Autodesk Fusion 360 part; units mm, degrees
note: some values were not read from the file. Set by a fixed rule: which sketch regions a step uses.
(part 2 of 2)
  line L93 (-6.3283, 34.4045) -> (-6.9169, 34.9918)
  spline S105 degree 3 poles (-6.9169, 34.9918) (-6.9414, 35.0193) (-6.976, 35.0359) (-7.0129, 35.0377) knots 0 0 0 0 1 1 1 1
  spline S106 degree 3 poles (-7.0129, 35.0377) (-7.0497, 35.0395) (-7.0858, 35.0264) (-7.1129, 35.0014) knots 0 0 0 0 1 1 1 1
  spline S107 degree 3 poles (-7.1129, 35.0014) (-7.1163, 34.9983) (-7.1195, 34.9951) (-7.1225, 34.9918) knots 0 0 0 0 1 1 1 1
  spline S108 degree 3 poles (-7.1225, 34.9918) (-7.1791, 34.9347) (-7.1791, 34.8426) (-7.1225, 34.7855) knots 0 0 0 0 1 1 1 1
  line L94 (-7.1225, 34.7855) -> (-6.428, 34.0972)
  spline S109 degree 3 poles (-6.428, 33.3938) (-6.4035, 33.3662) (-6.3689, 33.3497) (-6.3321, 33.3478) knots 0 0 0 0 1 1 1 1
  spline S110 degree 3 poles (-6.3321, 33.3478) (-6.2952, 33.346) (-6.2592, 33.3591) (-6.2321, 33.3841) knots 0 0 0 0 1 1 1 1
  spline S111 degree 3 poles (-6.2321, 33.3841) (-6.2287, 33.3872) (-6.2255, 33.3904) (-6.2224, 33.3938) knots 0 0 0 0 1 1 1 1
  line L95 (-6.2224, 33.3938) -> (-5.5348, 34.0862)
  spline S112 degree 3 poles (-5.5348, 34.0862) (-5.5068, 34.1107) (-5.49, 34.1456) (-5.4882, 34.1828) knots 0 0 0 0 1 1 1 1
  spline S113 degree 3 poles (-5.4882, 34.1828) (-5.4864, 34.22) (-5.4997, 34.2563) (-5.5252, 34.2835) knots 0 0 0 0 1 1 1 1
  spline S114 degree 3 poles (-5.5252, 34.2835) (-5.5282, 34.2869) (-5.5314, 34.2901) (-5.5348, 34.2931) knots 0 0 0 0 1 1 1 1
  spline S115 degree 3 poles (-5.5348, 34.2931) (-5.5622, 34.3198) (-5.5991, 34.3344) (-5.6373, 34.3337) knots 0 0 0 0 1 1 1 1
  spline S116 degree 3 poles (-5.6373, 34.3337) (-5.6755, 34.3337) (-5.7124, 34.3192) (-5.7404, 34.2931) knots 0 0 0 0 1 1 1 1
  line L96 (-5.7404, 34.2931) -> (-6.3166, 33.7066)
  line L97 (-6.3166, 33.7066) -> (-6.9032, 34.2931)
  spline S117 degree 3 poles (-6.9032, 34.2931) (-6.9304, 34.3207) (-6.9675, 34.3362) (-7.0063, 34.3362) knots 0 0 0 0 1 1 1 1
  spline S118 degree 3 poles (-7.0063, 34.3362) (-7.045, 34.3362) (-7.0822, 34.3207) (-7.1094, 34.2931) knots 0 0 0 0 1 1 1 1
  spline S119 degree 3 poles (-7.1094, 34.2931) (-7.1653, 34.2357) (-7.1653, 34.1443) (-7.1094, 34.0869) knots 0 0 0 0 1 1 1 1
  line L98 (-7.1094, 34.0869) -> (-6.428, 33.3938)
  spline S120 degree 3 poles (-8.3712, 34.8584) (-8.3467, 34.8308) (-8.3121, 34.8143) (-8.2752, 34.8124) knots 0 0 0 0 1 1 1 1
  spline S121 degree 3 poles (-8.2752, 34.8124) (-8.2384, 34.8106) (-8.2023, 34.8237) (-8.1752, 34.8487) knots 0 0 0 0 1 1 1 1
  line L99 (-8.1752, 34.8487) -> (-8.1656, 34.8584)
  line L100 (-8.1656, 34.8584) -> (-7.478, 35.546)
  spline S122 degree 3 poles (-7.478, 35.546) (-7.45, 35.5705) (-7.4332, 35.6054) (-7.4314, 35.6426) knots 0 0 0 0 1 1 1 1
  spline S123 degree 3 poles (-7.4314, 35.6426) (-7.4296, 35.6798) (-7.4429, 35.7161) (-7.4684, 35.7433) knots 0 0 0 0 1 1 1 1
  spline S124 degree 3 poles (-7.4684, 35.7433) (-7.4712, 35.7469) (-7.4745, 35.7501) (-7.478, 35.7529) knots 0 0 0 0 1 1 1 1
  spline S125 degree 3 poles (-7.478, 35.7529) (-7.5022, 35.7804) (-7.5363, 35.797) (-7.5729, 35.7992) knots 0 0 0 0 1 1 1 1
  spline S126 degree 3 poles (-7.5729, 35.7992) (-7.6094, 35.8014) (-7.6453, 35.789) (-7.6726, 35.7646) knots 0 0 0 0 1 1 1 1
  line L101 (-7.6726, 35.7646) -> (-7.6836, 35.7529)
  line L102 (-7.6836, 35.7529) -> (-8.2722, 35.1664)
  line L103 (-8.2722, 35.1664) -> (-8.8553, 35.7591)
  spline S127 degree 3 poles (-8.8553, 35.7591) (-8.8823, 35.7863) (-8.9194, 35.801) (-8.9577, 35.7997) knots 0 0 0 0 1 1 1 1
  spline S128 degree 3 poles (-8.9577, 35.7997) (-8.9962, 35.8005) (-9.0333, 35.7859) (-9.0609, 35.7591) knots 0 0 0 0 1 1 1 1
  spline S129 degree 3 poles (-9.0609, 35.7591) (-9.1175, 35.7063) (-9.1212, 35.6178) (-9.0691, 35.5604) knots 0 0 0 0 1 1 1 1
  line L104 (-9.0691, 35.5604) -> (-9.0609, 35.5522)
  line L105 (-9.0609, 35.5522) -> (-8.3712, 34.8584)
  spline S130 degree 3 poles (-8.3712, 34.0972) (-8.3467, 34.0696) (-8.3121, 34.0531) (-8.2752, 34.0513) knots 0 0 0 0 1 1 1 1
  spline S131 degree 3 poles (-8.2752, 34.0513) (-8.2384, 34.0495) (-8.2023, 34.0625) (-8.1752, 34.0875) knots 0 0 0 0 1 1 1 1
  spline S132 degree 3 poles (-8.1752, 34.0875) (-8.1724, 34.0911) (-8.1691, 34.0943) (-8.1656, 34.0972) knots 0 0 0 0 1 1 1 1
  line L106 (-8.1656, 34.0972) -> (-7.478, 34.7889)
  spline S133 degree 3 poles (-7.478, 34.7889) (-7.45, 34.8135) (-7.4332, 34.8483) (-7.4314, 34.8855) knots 0 0 0 0 1 1 1 1
  spline S134 degree 3 poles (-7.4314, 34.8855) (-7.4296, 34.9227) (-7.4429, 34.9591) (-7.4684, 34.9863) knots 0 0 0 0 1 1 1 1
  spline S135 degree 3 poles (-7.4684, 34.9863) (-7.4714, 34.9896) (-7.4746, 34.9928) (-7.478, 34.9959) knots 0 0 0 0 1 1 1 1
  spline S136 degree 3 poles (-7.478, 34.9959) (-7.5047, 35.0228) (-7.5411, 35.038) (-7.5791, 35.038) knots 0 0 0 0 1 1 1 1
  spline S137 degree 3 poles (-7.5791, 35.038) (-7.617, 35.038) (-7.6534, 35.0228) (-7.6802, 34.9959) knots 0 0 0 0 1 1 1 1
  line L107 (-7.6802, 34.9959) -> (-7.6836, 34.9959)
  line L108 (-7.6836, 34.9959) -> (-8.2722, 34.4087)
  line L109 (-8.2722, 34.4087) -> (-8.8553, 34.9959)
  spline S138 degree 3 poles (-8.8553, 34.9959) (-8.8822, 35.0233) (-8.9193, 35.0383) (-8.9577, 35.0371) knots 0 0 0 0 1 1 1 1
  spline S139 degree 3 poles (-8.9577, 35.0371) (-8.9962, 35.0377) (-9.0334, 35.0228) (-9.0609, 34.9959) knots 0 0 0 0 1 1 1 1
  spline S140 degree 3 poles (-9.0609, 34.9959) (-9.0888, 34.9713) (-9.1057, 34.9364) (-9.1075, 34.8992) knots 0 0 0 0 1 1 1 1
  spline S141 degree 3 poles (-9.1075, 34.8992) (-9.1093, 34.8621) (-9.096, 34.8257) (-9.0705, 34.7985) knots 0 0 0 0 1 1 1 1
  line L110 (-9.0705, 34.7985) -> (-9.0609, 34.7889)
  line L111 (-9.0609, 34.7889) -> (-8.3712, 34.0972)
  spline S142 degree 3 poles (-8.3712, 33.3938) (-8.3467, 33.3662) (-8.3121, 33.3497) (-8.2752, 33.3478) knots 0 0 0 0 1 1 1 1
  spline S143 degree 3 poles (-8.2752, 33.3478) (-8.2384, 33.346) (-8.2023, 33.3591) (-8.1752, 33.3841) knots 0 0 0 0 1 1 1 1
  spline S144 degree 3 poles (-8.1752, 33.3841) (-8.1722, 33.3875) (-8.169, 33.3907) (-8.1656, 33.3938) knots 0 0 0 0 1 1 1 1
  line L112 (-8.1656, 33.3938) -> (-7.478, 34.0862)
  spline S145 degree 3 poles (-7.478, 34.0862) (-7.4214, 34.1433) (-7.4214, 34.2354) (-7.478, 34.2925) knots 0 0 0 0 1 1 1 1
  spline S146 degree 3 poles (-7.478, 34.2925) (-7.5052, 34.32) (-7.5424, 34.3355) (-7.5811, 34.3355) knots 0 0 0 0 1 1 1 1
  spline S147 degree 3 poles (-7.5811, 34.3355) (-7.6199, 34.3355) (-7.657, 34.32) (-7.6843, 34.2925) knots 0 0 0 0 1 1 1 1
  line L113 (-7.6843, 34.2925) -> (-8.2729, 33.7059)
  line L114 (-8.2729, 33.7059) -> (-8.856, 34.2925)
  spline S148 degree 3 poles (-8.856, 34.2925) (-8.883, 34.3197) (-8.9201, 34.3344) (-8.9584, 34.333) knots 0 0 0 0 1 1 1 1
  spline S149 degree 3 poles (-8.9584, 34.333) (-8.9967, 34.3332) (-9.0336, 34.3187) (-9.0616, 34.2925) knots 0 0 0 0 1 1 1 1
  spline S150 degree 3 poles (-9.0616, 34.2925) (-9.0895, 34.2679) (-9.1064, 34.233) (-9.1082, 34.1958) knots 0 0 0 0 1 1 1 1
  spline S151 degree 3 poles (-9.1082, 34.1958) (-9.11, 34.1586) (-9.0966, 34.1223) (-9.0712, 34.0951) knots 0 0 0 0 1 1 1 1
  line L115 (-9.0712, 34.0951) -> (-9.0616, 34.0855)
  line L116 (-9.0616, 34.0855) -> (-8.3712, 33.3938)
  line L117 (-12.7412, 31.3041) -> (-12.7412, 31.2348)
  spline S152 degree 3 poles (-12.7412, 31.2348) (-12.6312, 31.2348) (-12.5602, 31.2117) (-12.5283, 31.1655) knots 0 0 0 0 1 1 1 1
  spline S153 degree 3 poles (-12.5283, 31.1655) (-12.4964, 31.1193) (-12.4805, 31.0148) (-12.4805, 30.8519) knots 0 0 0 0 1 1 1 1
  line L118 (-12.4805, 30.8519) -> (-12.4805, 30.3371)
  spline S154 degree 3 poles (-12.4805, 30.3371) (-12.5883, 30.4691) (-12.7236, 30.5351) (-12.8864, 30.5351) knots 0 0 0 0 1 1 1 1
  spline S155 degree 3 poles (-12.8864, 30.5351) (-13.0427, 30.5351) (-13.1769, 30.4757) (-13.2891, 30.3569) knots 0 0 0 0 1 1 1 1
  spline S156 degree 3 poles (-13.2891, 30.3569) (-13.4013, 30.238) (-13.4574, 30.095) (-13.4574, 29.9278) knots 0 0 0 0 1 1 1 1
  spline S157 degree 3 poles (-13.4574, 29.9278) (-13.4574, 29.7606) (-13.4013, 29.6181) (-13.2891, 29.5004) knots 0 0 0 0 1 1 1 1
  spline S158 degree 3 poles (-13.2891, 29.5004) (-13.1769, 29.3827) (-13.0427, 29.3238) (-12.8864, 29.3238) knots 0 0 0 0 1 1 1 1
  spline S159 degree 3 poles (-12.8864, 29.3238) (-12.7258, 29.3238) (-12.5894, 29.3909) (-12.4772, 29.5251) knots 0 0 0 0 1 1 1 1
  spline S160 degree 3 poles (-12.4772, 29.5251) (-12.4574, 29.4151) (-12.4409, 29.348) (-12.4277, 29.3238) knots 0 0 0 0 1 1 1 1
  line L119 (-12.4277, 29.3238) -> (-11.9854, 29.4063)
  line L120 (-11.9854, 29.4063) -> (-11.9854, 29.4756)
  spline S161 degree 3 poles (-11.9854, 29.4756) (-12.0954, 29.4756) (-12.1664, 29.4982) (-12.1983, 29.5433) knots 0 0 0 0 1 1 1 1
  spline S162 degree 3 poles (-12.1983, 29.5433) (-12.2302, 29.5884) (-12.2461, 29.6935) (-12.2461, 29.8585) knots 0 0 0 0 1 1 1 1
  line L121 (-12.2461, 29.8585) -> (-12.2461, 30.8519)
  spline S163 degree 3 poles (-12.2461, 30.8519) (-12.2461, 31.017) (-12.2302, 31.122) (-12.1983, 31.1671) knots 0 0 0 0 1 1 1 1
  spline S164 degree 3 poles (-12.1983, 31.1671) (-12.1664, 31.2123) (-12.0954, 31.2348) (-11.9854, 31.2348) knots 0 0 0 0 1 1 1 1
  line L122 (-11.9854, 31.2348) -> (-11.9854, 31.3041)
  line L123 (-11.9854, 31.3041) -> (-12.7412, 31.3041)
  spline S165 degree 3 poles (-12.8171, 30.4031) (-12.7423, 30.4031) (-12.6758, 30.3794) (-12.6174, 30.3321) knots 0 0 0 0 1 1 1 1
  spline S166 degree 3 poles (-12.6174, 30.3321) (-12.5591, 30.2848) (-12.5135, 30.2204) (-12.4805, 30.139) knots 0 0 0 0 1 1 1 1
  line L124 (-12.4805, 30.139) -> (-12.4805, 29.7133)
  spline S167 degree 3 poles (-12.4805, 29.7133) (-12.5135, 29.6341) (-12.5591, 29.5713) (-12.6174, 29.5251) knots 0 0 0 0 1 1 1 1
  spline S168 degree 3 poles (-12.6174, 29.5251) (-12.6758, 29.4789) (-12.7423, 29.4558) (-12.8171, 29.4558) knots 0 0 0 0 1 1 1 1
  spline S169 degree 3 poles (-12.8171, 29.4558) (-12.9381, 29.4558) (-13.0306, 29.4998) (-13.0944, 29.5878) knots 0 0 0 0 1 1 1 1
  spline S170 degree 3 poles (-13.0944, 29.5878) (-13.1582, 29.6759) (-13.1901, 29.7892) (-13.1901, 29.9278) knots 0 0 0 0 1 1 1 1
  spline S171 degree 3 poles (-13.1901, 29.9278) (-13.1901, 30.0664) (-13.1582, 30.1808) (-13.0944, 30.2711) knots 0 0 0 0 1 1 1 1
  spline S172 degree 3 poles (-13.0944, 30.2711) (-13.0306, 30.3591) (-12.9381, 30.4031) (-12.8171, 30.4031) knots 0 0 0 0 1 1 1 1
  spline S173 degree 3 poles (-14.441, 30.5351) (-14.6236, 30.5351) (-14.7804, 30.4757) (-14.9113, 30.3569) knots 0 0 0 0 1 1 1 1
  spline S174 degree 3 poles (-14.9113, 30.3569) (-15.0422, 30.238) (-15.1077, 30.095) (-15.1077, 29.9278) knots 0 0 0 0 1 1 1 1
  spline S175 degree 3 poles (-15.1077, 29.9278) (-15.1077, 29.7606) (-15.0417, 29.6187) (-14.9097, 29.502) knots 0 0 0 0 1 1 1 1
  spline S176 degree 3 poles (-14.9097, 29.502) (-14.7798, 29.3832) (-14.6236, 29.3238) (-14.441, 29.3238) knots 0 0 0 0 1 1 1 1
  spline S177 degree 3 poles (-14.441, 29.3238) (-14.2584, 29.3238) (-14.1016, 29.3827) (-13.9707, 29.5004) knots 0 0 0 0 1 1 1 1
  spline S178 degree 3 poles (-13.9707, 29.5004) (-13.8397, 29.6181) (-13.7743, 29.7606) (-13.7743, 29.9278) knots 0 0 0 0 1 1 1 1
  spline S179 degree 3 poles (-13.7743, 29.9278) (-13.7743, 30.095) (-13.8397, 30.238) (-13.9707, 30.3569) knots 0 0 0 0 1 1 1 1
  spline S180 degree 3 poles (-13.9707, 30.3569) (-14.1016, 30.4757) (-14.2584, 30.5351) (-14.441, 30.5351) knots 0 0 0 0 1 1 1 1
  spline S181 degree 3 poles (-14.441, 30.4064) (-14.3112, 30.4064) (-14.2121, 30.3613) (-14.1439, 30.2711) knots 0 0 0 0 1 1 1 1
  spline S182 degree 3 poles (-14.1439, 30.2711) (-14.0757, 30.1808) (-14.0416, 30.0664) (-14.0416, 29.9278) knots 0 0 0 0 1 1 1 1
  spline S183 degree 3 poles (-14.0416, 29.9278) (-14.0416, 29.7892) (-14.0757, 29.6748) (-14.1439, 29.5845) knots 0 0 0 0 1 1 1 1
  spline S184 degree 3 poles (-14.1439, 29.5845) (-14.2121, 29.4943) (-14.3112, 29.4492) (-14.441, 29.4492) knots 0 0 0 0 1 1 1 1
  spline S185 degree 3 poles (-14.441, 29.4492) (-14.5708, 29.4492) (-14.6698, 29.4938) (-14.738, 29.5829) knots 0 0 0 0 1 1 1 1
  spline S186 degree 3 poles (-14.738, 29.5829) (-14.8062, 29.672) (-14.8403, 29.787) (-14.8403, 29.9278) knots 0 0 0 0 1 1 1 1
  spline S187 degree 3 poles (-14.8403, 29.9278) (-14.8403, 30.0686) (-14.8062, 30.1841) (-14.738, 30.2744) knots 0 0 0 0 1 1 1 1
  spline S188 degree 3 poles (-14.738, 30.2744) (-14.6698, 30.3624) (-14.5708, 30.4064) (-14.441, 30.4064) knots 0 0 0 0 1 1 1 1
  line L125 (-15.913, 30.5384) -> (-16.1969, 29.776)
  line L126 (-16.1969, 29.776) -> (-16.5236, 30.5384)
  line L127 (-16.5236, 30.5384) -> (-16.5896, 30.5384)
  line L128 (-16.5896, 30.5384) -> (-16.923, 29.6407)
  spline S189 degree 3 poles (-16.923, 29.6407) (-16.9494, 29.568) (-16.9802, 29.5174) (-17.0154, 29.4888) knots 0 0 0 0 1 1 1 1
  spline S190 degree 3 poles (-17.0154, 29.4888) (-17.0506, 29.4602) (-17.0979, 29.4459) (-17.1573, 29.4459) knots 0 0 0 0 1 1 1 1
  line L129 (-17.1573, 29.4459) -> (-17.1573, 29.3799)
  line L130 (-17.1573, 29.3799) -> (-16.6952, 29.3799)
  line L131 (-16.6952, 29.3799) -> (-16.6952, 29.4459)
  spline S191 degree 3 poles (-16.6952, 29.4459) (-16.8053, 29.4459) (-16.8372, 29.5108) (-16.7909, 29.6407) knots 0 0 0 0 1 1 1 1
  line L132 (-16.7909, 29.6407) -> (-16.6127, 30.1555)
  line L133 (-16.6127, 30.1555) -> (-16.2761, 29.3799)
  line L134 (-16.2761, 29.3799) -> (-16.2035, 29.3799)
  line L135 (-16.2035, 29.3799) -> (-15.9361, 30.1555)
  line L136 (-15.9361, 30.1555) -> (-15.7117, 29.6407)
  spline S192 degree 3 poles (-15.7117, 29.6407) (-15.6545, 29.5108) (-15.6941, 29.4459) (-15.8305, 29.4459) knots 0 0 0 0 1 1 1 1
  line L137 (-15.8305, 29.4459) -> (-15.8305, 29.3799)
  line L138 (-15.8305, 29.3799) -> (-15.2331, 29.3799)
  line L139 (-15.2331, 29.3799) -> (-15.2331, 29.4459)
  spline S193 degree 3 poles (-15.2331, 29.4459) (-15.2837, 29.4459) (-15.3261, 29.4602) (-15.3602, 29.4888) knots 0 0 0 0 1 1 1 1
  spline S194 degree 3 poles (-15.3602, 29.4888) (-15.3943, 29.5174) (-15.4267, 29.568) (-15.4575, 29.6407) knots 0 0 0 0 1 1 1 1
  line L140 (-15.4575, 29.6407) -> (-15.847, 30.5384)
  line L141 (-15.847, 30.5384) -> (-15.913, 30.5384)
  spline S195 degree 3 poles (-17.8768, 30.5351) (-17.9692, 30.5351) (-18.0616, 30.5147) (-18.1541, 30.474) knots 0 0 0 0 1 1 1 1
  spline S196 degree 3 poles (-18.1541, 30.474) (-18.2465, 30.4333) (-18.3224, 30.3811) (-18.3818, 30.3173) knots 0 0 0 0 1 1 1 1
  line L142 (-18.3818, 30.3173) -> (-18.3224, 30.2447)
  spline S197 degree 3 poles (-18.3224, 30.2447) (-18.2762, 30.2887) (-18.2179, 30.325) (-18.1475, 30.3536) knots 0 0 0 0 1 1 1 1
  spline S198 degree 3 poles (-18.1475, 30.3536) (-18.0771, 30.3822) (-18.0143, 30.3965) (-17.9593, 30.3965) knots 0 0 0 0 1 1 1 1
  spline S199 degree 3 poles (-17.9593, 30.3965) (-17.7965, 30.3965) (-17.6793, 30.3453) (-17.6078, 30.243) knots 0 0 0 0 1 1 1 1
  spline S200 degree 3 poles (-17.6078, 30.243) (-17.5363, 30.1407) (-17.5105, 30.0081) (-17.5303, 29.8453) knots 0 0 0 0 1 1 1 1
  line L143 (-17.5303, 29.8453) -> (-18.3257, 29.8453)
  spline S201 degree 3 poles (-18.3257, 29.8453) (-18.3653, 29.7067) (-18.3378, 29.5851) (-18.2432, 29.4806) knots 0 0 0 0 1 1 1 1
  spline S202 degree 3 poles (-18.2432, 29.4806) (-18.1486, 29.3761) (-18.0264, 29.3238) (-17.8768, 29.3238) knots 0 0 0 0 1 1 1 1
  spline S203 degree 3 poles (-17.8768, 29.3238) (-17.7184, 29.3238) (-17.577, 29.3821) (-17.4527, 29.4987) knots 0 0 0 0 1 1 1 1
  spline S204 degree 3 poles (-17.4527, 29.4987) (-17.3284, 29.6154) (-17.2662, 29.7584) (-17.2662, 29.9278) knots 0 0 0 0 1 1 1 1
  spline S205 degree 3 poles (-17.2662, 29.9278) (-17.2662, 30.0972) (-17.3234, 30.2408) (-17.4379, 30.3585) knots 0 0 0 0 1 1 1 1
  spline S206 degree 3 poles (-17.4379, 30.3585) (-17.5523, 30.4762) (-17.6986, 30.5351) (-17.8768, 30.5351) knots 0 0 0 0 1 1 1 1
  line L144 (-18.098, 29.7232) -> (-17.5501, 29.7232)
  spline S207 degree 3 poles (-17.5501, 29.7232) (-17.5743, 29.6418) (-17.6144, 29.5768) (-17.6705, 29.5284) knots 0 0 0 0 1 1 1 1
  spline S208 degree 3 poles (-17.6705, 29.5284) (-17.7266, 29.48) (-17.7899, 29.4558) (-17.8603, 29.4558) knots 0 0 0 0 1 1 1 1
  spline S209 degree 3 poles (-17.8603, 29.4558) (-17.9593, 29.4558) (-18.0292, 29.485) (-18.0699, 29.5433) knots 0 0 0 0 1 1 1 1
  spline S210 degree 3 poles (-18.0699, 29.5433) (-18.1106, 29.6016) (-18.12, 29.6616) (-18.098, 29.7232) knots 0 0 0 0 1 1 1 1
  line L145 (-19.3819, 30.479) -> (-19.3819, 30.4097)
  spline S211 degree 3 poles (-19.3819, 30.4097) (-19.2718, 30.4097) (-19.2009, 30.3866) (-19.169, 30.3404) knots 0 0 0 0 1 1 1 1
  spline S212 degree 3 poles (-19.169, 30.3404) (-19.1371, 30.2942) (-19.1211, 30.1885) (-19.1211, 30.0235) knots 0 0 0 0 1 1 1 1
  line L146 (-19.1211, 30.0235) -> (-19.1211, 29.842)
  spline S213 degree 3 poles (-19.1211, 29.842) (-19.1211, 29.7254) (-19.1508, 29.6319) (-19.2102, 29.5614) knots 0 0 0 0 1 1 1 1
  spline S214 degree 3 poles (-19.2102, 29.5614) (-19.2696, 29.491) (-19.3246, 29.4558) (-19.3753, 29.4558) knots 0 0 0 0 1 1 1 1
  spline S215 degree 3 poles (-19.3753, 29.4558) (-19.4457, 29.4558) (-19.4809, 29.4921) (-19.4809, 29.5647) knots 0 0 0 0 1 1 1 1
  spline S216 degree 3 poles (-19.4809, 29.5647) (-19.4809, 29.5955) (-19.4924, 29.6231) (-19.5155, 29.6473) knots 0 0 0 0 1 1 1 1
  spline S217 degree 3 poles (-19.5155, 29.6473) (-19.5386, 29.6715) (-19.5656, 29.6836) (-19.5964, 29.6836) knots 0 0 0 0 1 1 1 1
  spline S218 degree 3 poles (-19.5964, 29.6836) (-19.6844, 29.6836) (-19.7284, 29.6319) (-19.7284, 29.5284) knots 0 0 0 0 1 1 1 1
  spline S219 degree 3 poles (-19.7284, 29.5284) (-19.7284, 29.48) (-19.7059, 29.4338) (-19.6607, 29.3898) knots 0 0 0 0 1 1 1 1
  spline S220 degree 3 poles (-19.6607, 29.3898) (-19.6156, 29.3458) (-19.5513, 29.3238) (-19.4677, 29.3238) knots 0 0 0 0 1 1 1 1
  spline S221 degree 3 poles (-19.4677, 29.3238) (-19.4017, 29.3238) (-19.3356, 29.3469) (-19.2696, 29.3931) knots 0 0 0 0 1 1 1 1
  spline S222 degree 3 poles (-19.2696, 29.3931) (-19.2036, 29.4393) (-19.1541, 29.4954) (-19.1211, 29.5614) knots 0 0 0 0 1 1 1 1
  spline S223 degree 3 poles (-19.1211, 29.5614) (-19.1035, 29.4448) (-19.0848, 29.3656) (-19.065, 29.3238) knots 0 0 0 0 1 1 1 1
  line L147 (-19.065, 29.3238) -> (-18.626, 29.4063)
  line L148 (-18.626, 29.4063) -> (-18.626, 29.4756)
  spline S224 degree 3 poles (-18.626, 29.4756) (-18.7361, 29.4756) (-18.807, 29.4987) (-18.8389, 29.5449) knots 0 0 0 0 1 1 1 1
  spline S225 degree 3 poles (-18.8389, 29.5449) (-18.8708, 29.5911) (-18.8868, 29.6957) (-18.8868, 29.8585) knots 0 0 0 0 1 1 1 1
  line L149 (-18.8868, 29.8585) -> (-18.8868, 30.0235)
  spline S226 degree 3 poles (-18.8868, 30.0235) (-18.8868, 30.1885) (-18.8708, 30.2942) (-18.8389, 30.3404) knots 0 0 0 0 1 1 1 1
  spline S227 degree 3 poles (-18.8389, 30.3404) (-18.807, 30.3866) (-18.7361, 30.4097) (-18.626, 30.4097) knots 0 0 0 0 1 1 1 1
  line L150 (-18.626, 30.4097) -> (-18.626, 30.479)
  line L151 (-18.626, 30.479) -> (-19.3819, 30.479)
  spline S228 degree 3 poles (-20.5667, 30.5351) (-20.6592, 30.5351) (-20.7516, 30.5147) (-20.844, 30.474) knots 0 0 0 0 1 1 1 1
  spline S229 degree 3 poles (-20.844, 30.474) (-20.9364, 30.4333) (-21.0123, 30.3811) (-21.0717, 30.3173) knots 0 0 0 0 1 1 1 1
  line L152 (-21.0717, 30.3173) -> (-21.0123, 30.2447)
  spline S230 degree 3 poles (-21.0123, 30.2447) (-20.9661, 30.2887) (-20.9078, 30.325) (-20.8374, 30.3536) knots 0 0 0 0 1 1 1 1
  spline S231 degree 3 poles (-20.8374, 30.3536) (-20.767, 30.3822) (-20.7043, 30.3965) (-20.6493, 30.3965) knots 0 0 0 0 1 1 1 1
  spline S232 degree 3 poles (-20.6493, 30.3965) (-20.4864, 30.3965) (-20.3693, 30.3453) (-20.2977, 30.243) knots 0 0 0 0 1 1 1 1
  spline S233 degree 3 poles (-20.2977, 30.243) (-20.2262, 30.1407) (-20.2004, 30.0081) (-20.2202, 29.8453) knots 0 0 0 0 1 1 1 1
  line L153 (-20.2202, 29.8453) -> (-21.0156, 29.8453)
  spline S234 degree 3 poles (-21.0156, 29.8453) (-21.0552, 29.7067) (-21.0277, 29.5851) (-20.9331, 29.4806) knots 0 0 0 0 1 1 1 1
  spline S235 degree 3 poles (-20.9331, 29.4806) (-20.8385, 29.3761) (-20.7164, 29.3238) (-20.5667, 29.3238) knots 0 0 0 0 1 1 1 1
  spline S236 degree 3 poles (-20.5667, 29.3238) (-20.4083, 29.3238) (-20.2669, 29.3821) (-20.1426, 29.4987) knots 0 0 0 0 1 1 1 1
  spline S237 degree 3 poles (-20.1426, 29.4987) (-20.0183, 29.6154) (-19.9561, 29.7584) (-19.9561, 29.9278) knots 0 0 0 0 1 1 1 1
  spline S238 degree 3 poles (-19.9561, 29.9278) (-19.9561, 30.0972) (-20.0134, 30.2408) (-20.1278, 30.3585) knots 0 0 0 0 1 1 1 1
  spline S239 degree 3 poles (-20.1278, 30.3585) (-20.2422, 30.4762) (-20.3885, 30.5351) (-20.5667, 30.5351) knots 0 0 0 0 1 1 1 1
  line L154 (-20.7879, 29.7232) -> (-20.24, 29.7232)
  spline S240 degree 3 poles (-20.24, 29.7232) (-20.2642, 29.6418) (-20.3043, 29.5768) (-20.3605, 29.5284) knots 0 0 0 0 1 1 1 1
  spline S241 degree 3 poles (-20.3605, 29.5284) (-20.4166, 29.48) (-20.4798, 29.4558) (-20.5502, 29.4558) knots 0 0 0 0 1 1 1 1
  spline S242 degree 3 poles (-20.5502, 29.4558) (-20.6493, 29.4558) (-20.7191, 29.485) (-20.7598, 29.5433) knots 0 0 0 0 1 1 1 1
  spline S243 degree 3 poles (-20.7598, 29.5433) (-20.8005, 29.6016) (-20.8099, 29.6616) (-20.7879, 29.7232) knots 0 0 0 0 1 1 1 1
  line L155 (-22.382, 30.5351) -> (-22.821, 30.4526)
  line L156 (-22.821, 30.4526) -> (-22.821, 30.3833)
  spline S244 degree 3 poles (-22.821, 30.3833) (-22.711, 30.3833) (-22.64, 30.3602) (-22.6081, 30.314) knots 0 0 0 0 1 1 1 1
  spline S245 degree 3 poles (-22.6081, 30.314) (-22.5762, 30.2678) (-22.5603, 30.1621) (-22.5603, 29.9971) knots 0 0 0 0 1 1 1 1
  line L157 (-22.5603, 29.9971) -> (-22.5603, 28.4426)
  line L158 (-22.5603, 28.4426) -> (-22.0652, 28.5251)
  line L159 (-22.0652, 28.5251) -> (-22.0652, 28.5944)
  spline S246 degree 3 poles (-22.0652, 28.5944) (-22.1752, 28.5944) (-22.2462, 28.6175) (-22.2781, 28.6637) knots 0 0 0 0 1 1 1 1
  spline S247 degree 3 poles (-22.2781, 28.6637) (-22.31, 28.7099) (-22.3259, 28.8155) (-22.3259, 28.9806) knots 0 0 0 0 1 1 1 1
  line L160 (-22.3259, 28.9806) -> (-22.3259, 29.5185)
  spline S248 degree 3 poles (-22.3259, 29.5185) (-22.2203, 29.3887) (-22.0861, 29.3238) (-21.9233, 29.3238) knots 0 0 0 0 1 1 1 1
  spline S249 degree 3 poles (-21.9233, 29.3238) (-21.767, 29.3238) (-21.6323, 29.3827) (-21.5189, 29.5004) knots 0 0 0 0 1 1 1 1
  spline S250 degree 3 poles (-21.5189, 29.5004) (-21.4056, 29.6181) (-21.349, 29.7606) (-21.349, 29.9278) knots 0 0 0 0 1 1 1 1
  spline S251 degree 3 poles (-21.349, 29.9278) (-21.349, 30.095) (-21.4056, 30.238) (-21.5189, 30.3569) knots 0 0 0 0 1 1 1 1
  spline S252 degree 3 poles (-21.5189, 30.3569) (-21.6323, 30.4757) (-21.767, 30.5351) (-21.9233, 30.5351) knots 0 0 0 0 1 1 1 1
  spline S253 degree 3 poles (-21.9233, 30.5351) (-22.0861, 30.5351) (-22.2214, 30.468) (-22.3292, 30.3338) knots 0 0 0 0 1 1 1 1
  spline S254 degree 3 poles (-22.3292, 30.3338) (-22.349, 30.435) (-22.3666, 30.5021) (-22.382, 30.5351) knots 0 0 0 0 1 1 1 1
  spline S255 degree 3 poles (-21.9926, 30.4031) (-21.8693, 30.4031) (-21.7758, 30.3591) (-21.712, 30.2711) knots 0 0 0 0 1 1 1 1
  spline S256 degree 3 poles (-21.712, 30.2711) (-21.6482, 30.183) (-21.6163, 30.0686) (-21.6163, 29.9278) knots 0 0 0 0 1 1 1 1
  spline S257 degree 3 poles (-21.6163, 29.9278) (-21.6163, 29.7892) (-21.6482, 29.6759) (-21.712, 29.5878) knots 0 0 0 0 1 1 1 1
  spline S258 degree 3 poles (-21.712, 29.5878) (-21.7758, 29.4998) (-21.8693, 29.4558) (-21.9926, 29.4558) knots 0 0 0 0 1 1 1 1
  spline S259 degree 3 poles (-21.9926, 29.4558) (-22.0652, 29.4558) (-22.1312, 29.4795) (-22.1906, 29.5268) knots 0 0 0 0 1 1 1 1
  spline S260 degree 3 poles (-22.1906, 29.5268) (-22.25, 29.5741) (-22.2951, 29.6374) (-22.3259, 29.7166) knots 0 0 0 0 1 1 1 1
  line L161 (-22.3259, 29.7166) -> (-22.3259, 30.1423)
  spline S261 degree 3 poles (-22.3259, 30.1423) (-22.2951, 30.2215) (-22.25, 30.2848) (-22.1906, 30.3321) knots 0 0 0 0 1 1 1 1
  spline S262 degree 3 poles (-22.1906, 30.3321) (-22.1312, 30.3794) (-22.0652, 30.4031) (-21.9926, 30.4031) knots 0 0 0 0 1 1 1 1
  line L162 (-23.9927, 30.5351) -> (-24.1379, 30.314)
  spline S263 degree 3 poles (-24.1379, 30.314) (-24.2413, 30.4614) (-24.3821, 30.5351) (-24.5604, 30.5351) knots 0 0 0 0 1 1 1 1
  spline S264 degree 3 poles (-24.5604, 30.5351) (-24.7166, 30.5351) (-24.8508, 30.4757) (-24.963, 30.3569) knots 0 0 0 0 1 1 1 1
  spline S265 degree 3 poles (-24.963, 30.3569) (-25.0752, 30.238) (-25.1314, 30.095) (-25.1314, 29.9278) knots 0 0 0 0 1 1 1 1
  spline S266 degree 3 poles (-25.1314, 29.9278) (-25.1314, 29.7606) (-25.0752, 29.6181) (-24.963, 29.5004) knots 0 0 0 0 1 1 1 1
  spline S267 degree 3 poles (-24.963, 29.5004) (-24.8508, 29.3827) (-24.7166, 29.3238) (-24.5604, 29.3238) knots 0 0 0 0 1 1 1 1
  spline S268 degree 3 poles (-24.5604, 29.3238) (-24.3975, 29.3238) (-24.2633, 29.3887) (-24.1577, 29.5185) knots 0 0 0 0 1 1 1 1
  line L163 (-24.1577, 29.5185) -> (-24.1577, 28.4426)
  line L164 (-24.1577, 28.4426) -> (-23.6626, 28.5251)
  line L165 (-23.6626, 28.5251) -> (-23.6626, 28.5944)
  spline S269 degree 3 poles (-23.6626, 28.5944) (-23.7726, 28.5944) (-23.8436, 28.6175) (-23.8755, 28.6637) knots 0 0 0 0 1 1 1 1
  spline S270 degree 3 poles (-23.8755, 28.6637) (-23.9074, 28.7099) (-23.9234, 28.8155) (-23.9234, 28.9806) knots 0 0 0 0 1 1 1 1
  line L166 (-23.9234, 28.9806) -> (-23.9234, 30.5351)
  line L167 (-23.9234, 30.5351) -> (-23.9927, 30.5351)
  spline S271 degree 3 poles (-24.4911, 30.4031) (-24.4162, 30.4031) (-24.3497, 30.3794) (-24.2914, 30.3321) knots 0 0 0 0 1 1 1 1
  spline S272 degree 3 poles (-24.2914, 30.3321) (-24.2331, 30.2848) (-24.1885, 30.2204) (-24.1577, 30.139) knots 0 0 0 0 1 1 1 1
  line L168 (-24.1577, 30.139) -> (-24.1577, 29.7166)
  spline S273 degree 3 poles (-24.1577, 29.7166) (-24.1885, 29.6374) (-24.2331, 29.5741) (-24.2914, 29.5268) knots 0 0 0 0 1 1 1 1
  spline S274 degree 3 poles (-24.2914, 29.5268) (-24.3497, 29.4795) (-24.4162, 29.4558) (-24.4911, 29.4558) knots 0 0 0 0 1 1 1 1
  spline S275 degree 3 poles (-24.4911, 29.4558) (-24.6143, 29.4558) (-24.7078, 29.4998) (-24.7716, 29.5878) knots 0 0 0 0 1 1 1 1
  spline S276 degree 3 poles (-24.7716, 29.5878) (-24.8354, 29.6759) (-24.8673, 29.7892) (-24.8673, 29.9278) knots 0 0 0 0 1 1 1 1
  spline S277 degree 3 poles (-24.8673, 29.9278) (-24.8673, 30.0686) (-24.8354, 30.183) (-24.7716, 30.2711) knots 0 0 0 0 1 1 1 1
  spline S278 degree 3 poles (-24.7716, 30.2711) (-24.7078, 30.3591) (-24.6143, 30.4031) (-24.4911, 30.4031) knots 0 0 0 0 1 1 1 1
  spline S279 degree 3 poles (-25.5637, 31.3701) (-25.6121, 31.3701) (-25.6528, 31.3294) (-25.6858, 31.248) knots 0 0 0 0 1 1 1 1
  line L169 (-25.6858, 31.248) -> (-26.3294, 29.6407)
  spline S280 degree 3 poles (-26.3294, 29.6407) (-26.3822, 29.5108) (-26.4604, 29.4459) (-26.5638, 29.4459) knots 0 0 0 0 1 1 1 1
  line L170 (-26.5638, 29.4459) -> (-26.5638, 29.3799)
  line L171 (-26.5638, 29.3799) -> (-26.1017, 29.3799)
  line L172 (-26.1017, 29.3799) -> (-26.1017, 29.4459)
  spline S281 degree 3 poles (-26.1017, 29.4459) (-26.1699, 29.4459) (-26.2106, 29.4597) (-26.2238, 29.4872) knots 0 0 0 0 1 1 1 1
  spline S282 degree 3 poles (-26.2238, 29.4872) (-26.237, 29.5147) (-26.2282, 29.5658) (-26.1974, 29.6407) knots 0 0 0 0 1 1 1 1
  line L173 (-26.1974, 29.6407) -> (-25.9862, 30.1687)
  line L174 (-25.9862, 30.1687) -> (-25.7452, 29.6407)
  spline S283 degree 3 poles (-25.7452, 29.6407) (-25.71, 29.5592) (-25.7001, 29.5064) (-25.7155, 29.4822) knots 0 0 0 0 1 1 1 1
  spline S284 degree 3 poles (-25.7155, 29.4822) (-25.7309, 29.458) (-25.7761, 29.4459) (-25.8509, 29.4459) knots 0 0 0 0 1 1 1 1
  line L175 (-25.8509, 29.4459) -> (-25.8509, 29.3799)
  line L176 (-25.8509, 29.3799) -> (-25.2667, 29.3799)
  line L177 (-25.2667, 29.3799) -> (-25.2667, 29.4459)
  spline S285 degree 3 poles (-25.2667, 29.4459) (-25.3173, 29.4459) (-25.358, 29.4597) (-25.3888, 29.4872) knots 0 0 0 0 1 1 1 1
  spline S286 degree 3 poles (-25.3888, 29.4872) (-25.4196, 29.5147) (-25.4526, 29.5658) (-25.4878, 29.6407) knots 0 0 0 0 1 1 1 1
  line L178 (-25.4878, 29.6407) -> (-25.8674, 30.4625)
  line L179 (-25.8674, 30.4625) -> (-25.7023, 30.875)
  spline S287 degree 3 poles (-25.7023, 30.875) (-25.6737, 30.9477) (-25.638, 31.0076) (-25.5951, 31.0549) knots 0 0 0 0 1 1 1 1
  spline S288 degree 3 poles (-25.5951, 31.0549) (-25.5522, 31.1022) (-25.5175, 31.1396) (-25.4911, 31.1671) knots 0 0 0 0 1 1 1 1
  spline S289 degree 3 poles (-25.4911, 31.1671) (-25.4647, 31.1946) (-25.4515, 31.226) (-25.4515, 31.2612) knots 0 0 0 0 1 1 1 1
  spline S290 degree 3 poles (-25.4515, 31.2612) (-25.4515, 31.2986) (-25.4631, 31.3261) (-25.4862, 31.3437) knots 0 0 0 0 1 1 1 1
  spline S291 degree 3 poles (-25.4862, 31.3437) (-25.5093, 31.3613) (-25.5351, 31.3701) (-25.5637, 31.3701) knots 0 0 0 0 1 1 1 1
extrude "Extrude7" cut sketch "Sketch10" against normal blind 1 contours L18 L19 L20 S0 S1 L21 L22 L23 S2 S3 L24 L25 L26 L27 L28 S4 S5 S6 S7 | L29 S8 S9 S10 S11 S12 S13 L30 S14 S15 | L33 L34 L35 S19 S20 S21 S22 L36 L37 | L39 L40 L41 S27 S28 S29 S30 L42 L43 | S35 S36 S37 S38 S39 | L44 L45 L46 L47 L48 L49 L50 L51 L52 L53 L54 L55 L56 | L62 S51 S52 S54 S55 L65 | L57 S44 S45 L58 S46 S47 L59 L60 L61 L62 S54 S55 L65 | L59 S48 S49 S50 L60 L62 S51 S52 S53 L63 L64 L65 S56 S57 L66 S58 S59 | L59 S48 S49 S50 L60 L65 | S60 S61 L67 L68 S62 S63 S64 S65 S66 L69 L70 L71 S67 S68 S69 L72 L73 | S70 S71 L74 L75 S72 S73 S74 S75 S76 S77 L76 L77 S78 S79 S80 L78 L79 | S81 S82 L80 L81 S83 S84 S85 L82 L83 S86 S87 S88 L84 L85 | S89 S90 S91 L86 S92 S93 S94 S95 S96 L87 L88 S97 S98 S99 L89 | S100 S101 L90 L91 S102 S103 S104 L92 L93 S105 S106 S107 S108 L94 | S109 S110 S111 L95 S112 S113 S114 S115 S116 L96 L97 S117 S118 S119 L98 | S120 S121 L99 L100 S122 S123 S124 S125 S126 L101 L102 L103 S127 S128 S129 L104 L105 | S130 S131 S132 L106 S133 S134 S135 S136 S137 L107 L108 L109 S138 S139 S140 S141 L110 L111 | S142 S143 S144 L112 S145 S146 S147 L113 L114 S148 S149 S150 S151 L115 L116 bodies 6 in component "GNSS_Enclosure_Top"
component "GNSS_PCB" placed x (1, 0, 0) y (0, 1, 0) z (0, 0, 1) at (0, 0, 0)
component "GNSS_Enclosure_Bottom" placed x (1, 0, 0) y (0, 1, 0) z (0, 0, 1) at (0, 0, 0)
component "GNSS_Enclosure_Top" placed x (1, 0, 0) y (0, 1, 0) z (0, 0, 1) at (0, 0, 0)
equation "PCB_X_Size = 100 mm"
equation "PCB_Y_Size = 75 mm"
equation "PCB_Bolt_Inset = 2.5 mm"
equation "PCB_Z_Size = 1.7 mm"
equation "d6 = PCB_Y_Size + ( PCB_Y_Size * PCB_Shrinkage_Percent )"
equation "PCB_Shrinkage_Percent = 0.00"
equation "d8 = PCB_X_Size + ( PCB_X_Size * PCB_Shrinkage_Percent )"
equation "d9 = PCB_Bolt_Inset"
equation "d10 = PCB_Bolt_Inset"
equation "Screen_PCB_X_Size = 61 mm"
equation "Screen_PCB_Y_Size = 39.5 mm"
equation "Screen_DisplayArea_X_Size = 49.5 mm"
equation "Screen_DisplayArea_Y_Size = 25.5 mm"
equation "Screen_DisplayArea_X_Offset = 3 mm"
equation "Screen_DisplayArea_Y_Offset = 7.5 mm"
equation "Screen_Center_X_Offset = 0 mm"
equation "Screen_Center_Y_Offset = -11.325 mm"
equation "d19 = Screen_PCB_X_Size"
equation "d20 = Screen_PCB_Y_Size"
equation "d21 = ( Screen_PCB_X_Size / 2 ) + Screen_Center_X_Offset"
equation "d22 = ( Screen_PCB_Y_Size / 2 ) + Screen_Center_Y_Offset"
equation "d23 = Screen_DisplayArea_X_Size"
equation "d24 = Screen_DisplayArea_Y_Size"
equation "d25 = ( Screen_PCB_Y_Size - Screen_DisplayArea_Y_Size ) / 2"
equation "d26 = Screen_DisplayArea_X_Offset"
equation "BatteryHolder_X_Size = 77 mm"
equation "BatteryHolder_Y_Size = 20.65 mm"
equation "BatteryHolder_Z_Size = 18.5 mm"
equation "d30 = BatteryHolder_X_Size"
equation "d31 = BatteryHolder_Y_Size"
equation "d32 = ( BatteryHolder_X_Size / 2 ) + BatteryHolder_Center_X_Offset"
equation "BatteryHolder_Center_X_Offset = 0 mm"
equation "BatteryHolder_Center_Y_Offset = 25.5 mm"
equation "d35 = ( BatteryHolder_Y_Size / 2 ) + BatteryHolder_Center_Y_Offset"
equation "USB_X_Center_Offset = 17 mm"
equation "SolarInput_X_CenterOffset = 10 mm"
equation "d38 = USB_X_Center_Offset"
equation "d39 = SolarInput_X_CenterOffset"
equation "USB_Jack_X_Size = 9 mm"
equation "USB_Jack_Z_Size = 3.4 mm"
equation "USB_Jack_Y_Size = 7.4 mm"
equation "d43 = USB_Jack_X_Size"
equation "d44 = USB_Jack_Y_Size"
equation "d45 = USB_Jack_Y_Size"
equation "SolarInput_X_Size = 5.5 mm"
equation "SolarInput_Y_Size = 12 mm"
equation "SolarInput_Z_Size = 8.5 mm"
equation "d49 = SolarInput_X_Size"
equation "d50 = SolarInput_Y_Size"
equation "d51 = SolarInput_Y_Size - SolarInput_EdgeOverhang"
equation "SolarInput_EdgeOverhang = 3 mm"
equation "Antenna_PCB_Center_Offset = -4 mm"
equation "d54 = -Antenna_PCB_Center_Offset"
equation "d55 = PCB_Z_Size"
equation "d57 = BatteryHolder_Z_Size"
equation "d59 = SolarInput_Z_Size"
equation "d62 = BatteryHolder_Y_Size / 2"
equation "d64 = BatteryHolder_Y_Size / 2"
equation "d65 = PCB_Z_Size + 0.2 mm"
equation "d66 = USB_Jack_Z_Size"
equation "Screen_Z_Offset = 11 mm"
equation "d69 = Screen_Z_Offset"
equation "d70 = PCB_Z_Size"
equation "Screen_Display_Z_Size = 1.3 mm"
equation "Screen_Y_Size = 29.2 mm"
equation "d74 = Screen_PCB_X_Size"
equation "d75 = Screen_Y_Size"
equation "d76 = ( Screen_PCB_Y_Size - Screen_Y_Size ) / 2"
equation "d77 = Screen_Display_Z_Size"
equation "d80 = PCB_Bolt_Hole_Diameter"
equation "PCB_Bolt_Hole_Diameter = 2.1 mm"
equation "Enclosure_Wall_Thickness = 2 mm"
equation "PCB_Bottom_Z_Clearance = 3 mm"
equation "d85 = -PCB_Bottom_Z_Clearance"
equation "PCB_Horizontal_Clearance = 1 mm"
equation "d87 = PCB_Horizontal_Clearance"
equation "d88 = PCB_Horizontal_Clearance + Enclosure_Wall_Thickness"
equation "d89 = -Enclosure_Wall_Thickness"
equation "d95 = PCB_Bottom_Z_Clearance"
equation "d98 = Heatset_Insert_Hole_Size"
equation "Cutout_Clearance = 1 mm"
equation "d102 = Cutout_Clearance"
equation "USB_C_Plug_X_Size = 14 mm"
equation "USB_C_Plug_Y_Size = 10 mm"
equation "d107 = USB_C_Plug_X_Size"
equation "d108 = USB_C_Plug_Y_Size"
equation "d112 = d111"
equation "d113 = Enclosure_Wall_Thickness"
equation "d115 = Enclosure_Wall_Thickness"
equation "Battery_Ceiling_Clearance = 2 mm"
equation "d117 = -Battery_Ceiling_Clearance"
equation "d120 = Enclosure_Wall_Thickness"
equation "Antenna_Hole_Diameter = 10 mm"
equation "Antenna_PCB_Center_Z_Offset = 6.5 mm"
equation "d124 = Antenna_PCB_Center_Z_Offset + PCB_Z_Size"
equation "d126 = Antenna_Hole_Diameter"
equation "Enclosure_Bolt_Flange_Diameter = 6 mm"
equation "d129 = Enclosure_Bolt_Flange_Diameter"
equation "d130 = Enclosure_Bolt_Flange_Diameter"
equation "d131 = Enclosure_Bolt_Flange_Diameter * 2"
equation "d132 = d131"
equation "d133 = d131"
equation "d134 = d131"
equation "d137 = Enclosure_Bolt_Flange_Diameter / 2"
equation "d139 = Heatset_Insert_Hole_Size"
equation "d159 = Enclosure_Wall_Thickness"
equation "d160 = Enclosure_Chamfer"
equation "Enclosure_Chamfer = 1 mm"
equation "d162 = Enclosure_Chamfer"
equation "Heatset_Insert_Hole_Size = 3 mm"
